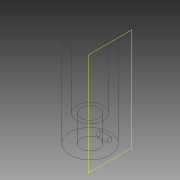
# Autodesk Inventor part: Screw_Asm_Jig_Upper
Saved by Autodesk Inventor 2011 SP2 (Build 150309200, 309)
## iProperties
Created: 2012-02-15
Part Number: Screw_Asm_Jig_Upper
Document SubType Name: Modeling
Designer: sungwook
Density: 1 g/cm^3
Author: sungwook
Autodesk Inventor part; units mm, degrees
ref_plane "XZ Plane" through (0, 0, 0) normal (0, 1, 0) x (-1, 0, 0)
ref_plane "XY Plane" through (0, 0, 0) normal (0, 0, 1) x (1, 0, 0)
sketch "Sketch1" plane through (0, 0, 0) normal (0, 0, 1) x (1, 0, 0)
  circle A0 centre (0, 0) radius 7.5
  dimension "d0" = 15
  constraints: 1 centre point, 1 coincident
  measures "d0" diameter of A0
extrude "Extrusion1" add sketch "Sketch1" along normal blind 35
hole "Hole1" at (0, 0, 0) direction (0, 0, 1) diameter 6.785 end through all
hole "Hole2" at (0, 0, 35) direction (0, 0, -1) diameter 10 depth 25
chamfer "Chamfer1" distance 0.5 angle 45 1 edges at (-7.5, 0, 35)
ref_plane "Work Plane1" through (7.5, 0, 0) normal (1, 0, 0) x (0, 1, 0)
sketch "Sketch2" plane through (7.5, 0, 0) normal (1, 0, 0) x (0, 1, 0)
  line L0 (-7.5, 0) -> (-7.5, 34.5) projected
  line L1 (-3.3925, 10) -> (-3.3925, 0) projected
  line L2 (3.3925, 10) -> (3.3925, 0) projected
  line L3 (-7.5, 0) -> (7.5, 0) projected
  line L4 (5, 10) -> (-5, 10) projected
  line L5 (0, -7) -> (0, 42) projected
  point P0 (0, 0)
  point P1 (0, 5)
  dimension "d24" = 5
  dimension "d25" = 5
  constraints: 1 point on line
  measures "d24" distance from line of point (0, 5) L4
  measures "d25" distance of point (0, 5) point (0, 0)
hole "Hole3" at (7.5, 0, 5) direction (-1, 0, 0) diameter 1.694 depth 7.5 thread size "2-56 UNC" class "2B" standard "ANSI Unified Screw Threads"
body "Solid1"
